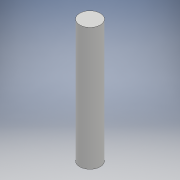
# Autodesk Inventor part: Палец
Saved by Autodesk Inventor 2018 (Build 220112000, 112)
## iProperties
Created: 2018-11-12
Part Number: Палец
Material: Типовые
Document SubType Name: Modeling
Designer: Lev
Density: 1 g/cm^3
Appearance: По умолчанию
Author: Lev
Autodesk Inventor part; units mm, degrees
ref_plane "YZ Plane" through (0, 0, 0) normal (1, 0, 0) x (0, 1, 0)
ref_plane "XZ Plane" through (0, 0, 0) normal (0, 1, 0) x (-1, 0, 0)
ref_plane "XY Plane" through (0, 0, 0) normal (0, 0, 1) x (1, 0, 0)
sketch "Эскиз1" plane through (0, 0, 0) normal (0, 0, 1) x (1, 0, 0)
  circle A0 centre (0, 0) radius 2.5
  dimension "d0" = 5
  constraints: 1 centre point, 1 coincident
  measures "d0" diameter of A0
extrude "Выдавливание1" add sketch "Эскиз1" along normal mid plane 30
